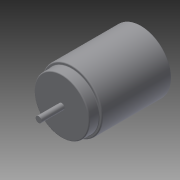
# Autodesk Inventor part: Motor
Saved by Autodesk Inventor 2015 (Build 190159000, 159)
## iProperties
Created: 2018-02-28
Part Number: Motor
Material: Generic
Document SubType Name: Modeling
Designer: Administrator
Density: 1 g/cm^3
Appearance: Default
Author: Administrator
Autodesk Inventor part; units mm, degrees
ref_plane "YZ Plane" through (0, 0, 0) normal (1, 0, 0) x (0, 1, 0)
ref_plane "XZ Plane" through (0, 0, 0) normal (0, 1, 0) x (-1, 0, 0)
ref_plane "XY Plane" through (0, 0, 0) normal (0, 0, 1) x (1, 0, 0)
sketch "Sketch1" plane through (0, 0, 0) normal (0, 0, 1) x (1, 0, 0)
  circle A0 centre (0, 0) radius 1.016
  circle A1 centre (0, 0) radius 10.414
  dimension "d0" = 2.032
  dimension "d1" = 20.828
  constraints: 2 centre point, 2 coincident
  measures "d0" diameter of A0
  measures "d1" diameter of A1
extrude "Extrusion1" add sketch "Sketch1" along normal blind 7.874 contours A0
extrude "Extrusion2" add sketch "Sketch1" against normal blind 27.305 contours A0 | A1
sketch "Sketch2" plane through (0, 0, 0) normal (0, 0, 1) x (1, 0, 0)
  circle A0 centre (0, 0) radius 9.4615
  circle A1 centre (0, 0) radius 10.414
  dimension "d6" = 18.923
  constraints: 2 centre point, 2 coincident
  measures "d6" diameter of A0
extrude "Extrusion3" cut sketch "Sketch2" against normal blind 3.429
fillet "Fillet1" radius 0.3556 3 edges at (-9.4615, 0, 0) (-10.414, 0, -3.429) (-10.414, 0, -27.305)
fillet "Fillet2" radius 0.1778 1 edges at (-9.4615, 0, -3.429)
body "Solid1"
